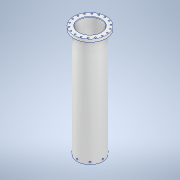
# Autodesk Inventor part: ODSY-0003-401
Saved by Autodesk Inventor 2021 (Build 250183000, 183)
## iProperties
Created: 2021-10-28
Part Number: ODSY-0003-401
Project: ODYSSEY
Material: Aluminum 6061
Description: COMBUSTION CHAMBER FINAL DIMENSIONS
Document SubType Name: Modeling
Designer: ALEX CLAY
Density: 2.7 g/cm^3
Appearance: Aluminum - Flat
Mass: 3091.69 g
Surface Area: 3602.64 cm^2
Volume: 1145.07 cm^3
Author: ALEX CLAY
Revision Number: 00
Autodesk Inventor part; units mm, degrees
note: some values were not read from the file. Chosen so that the rebuilt part matches the saved one: direction of "Hole2".
ref_plane "YZ Plane" through (0, 0, 0) normal (1, 0, 0) x (0, 1, 0)
ref_plane "XZ Plane" through (0, 0, 0) normal (0, 1, 0) x (-1, 0, 0)
sketch "Sketch1" plane through (0, 0, 0) normal (0, 1, 0) x (-1, 0, 0)
  circle A0 centre (0, 0) radius 50.8
  circle A1 centre (0, 0) radius 57.15
  dimension "d0" = 114.3
  dimension "d1" = 101.6
  constraints: 2 centre point, 2 coincident
  measures "d0" diameter of A1
  measures "d1" diameter of A0
extrude "Extrusion1" add sketch "Sketch1" along normal blind 498.475
sketch "Sketch2" plane through (0, 498.475, 0) normal (0, 1, 0) x (1, 0, 0)
  circle A0 centre (0, 0) radius 73.025
  circle A1 centre (0, 0) radius 57.15
  circle A2 centre (0, 0) radius 57.15 projected
  dimension "d4" = 146.05
  constraints: 2 centre point, 2 coincident, 1 concentric
  measures "d4" diameter of A0
extrude "Extrusion2" add sketch "Sketch2" against normal blind 12.7
sketch "Sketch3" plane through (0, 498.475, 0) normal (0, 1, 0) x (1, 0, 0)
  point P0 (0, 0)
  point P1 (0, -66.675)
  dimension "d7" = 66.675
  constraints: 1 vertical alignment
  measures "d7" distance of point (0, -66.675) point (0, 0)
hole "Hole1" at (0, 498.475, 66.675) direction (0, -1, 0) diameter 6.7564 end through all clearance for "Socket Head Cap Screw" size "1/4" standard "Ansi Unified Screw Threads"
pattern_circular "Circular Pattern1" count 18 over 360 about axis through (0, 0, 0) along (0, 1, 0) of "Hole1"
chamfer "Chamfer1" distance 3.175 angle 15 1 edges at (50.8, 498.475, 0) measured on face at (13.148, 332.3167, -49.069)
chamfer "Chamfer2" distance 3.175 angle 15 1 edges at (50.8, 0, 0) measured on face at (-25.4, 330.2, -43.9941)
ref_plane "Work Plane1" through (0, 0, 57.15) normal (0, 0, 1) x (1, 0, 0)
sketch "Sketch4" plane through (0, 0, 57.15) normal (0, 0, 1) x (1, 0, 0)
  point P0 (0, 0)
  point P1 (0, 10.16)
  dimension "d24" = 10.16
  constraints: 1 vertical alignment
  measures "d24" distance of point (0, 0) point (0, 10.16)
hole "Hole2" at (0, 10.16, 57.15) direction (0, 0, -1) diameter 6.7564 end up to surface clearance for "Socket Head Cap Screw" size "1/4" standard "Ansi Unified Screw Threads"
pattern_circular "Circular Pattern2" count 8 over 360 about axis through (0, 0, 0) along (0, 1, 0) of "Hole2"
body "Solid1"
